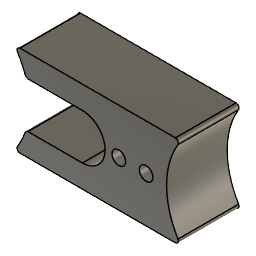
CUERPOMESA (Autodesk Fusion 360 design; units mm, degrees)
part number: 2026-05-18-09-44-16-687
Autodesk Fusion 360 part; units mm, degrees
sketch "Boceto2" plane through (0, 0, 0) normal (0, 1, 0) x (1, 0, 0)
  line L0 (-36.936, 0) -> (-1061.822, 0)
  line L1 (-1061.822, -600) -> (-36.936, -600)
  line L2 (-1008.5735, -150) -> (-650, -150)
  line L3 (-650, -450) -> (-1008.5735, -450)
  arc A0 (-1078.675, -569.2308) -> (-1027.4745, -463.4615) centre (-1500, -300) ccw
  arc A1 (-1027.4745, -136.5385) -> (-1078.675, -30.7692) centre (-1500, -300) ccw
  arc A2 (-650, -450) -> (-500, -300) centre (-650, -300) ccw
  arc A3 (-500, -300) -> (-650, -150) centre (-650, -300) ccw
  circle A4 centre (-410, -300) radius 45
  circle A5 centre (-230, -300) radius 45
  arc A6 (-19.821, -30.3477) -> (-19.821, -569.6523) centre (426.1842, -300) ccw
  arc A7 (-1078.675, -569.2308) -> (-1061.822, -600) centre (-1061.822, -580) ccw
  arc A8 (-36.936, -600) -> (-19.821, -569.6523) centre (-36.936, -580) ccw
  arc A9 (-19.821, -30.3477) -> (-36.936, 0) centre (-36.936, -20) ccw
  arc A10 (-1061.822, 0) -> (-1078.675, -30.7692) centre (-1061.822, -20) ccw
  arc A11 (-1027.4745, -136.5385) -> (-1008.5735, -150) centre (-1008.5735, -130) ccw
  arc A12 (-1008.5735, -450) -> (-1027.4745, -463.4615) centre (-1008.5735, -470) ccw
  point P0 (-1100, 0)
  point P1 (0, -600)
  point P2 (-500, -150)
  point P3 (-500, -450)
  dimension "d1" = 1100
  dimension "d2" = 600
  dimension "d6" = 300
  dimension "d13" = 150
  dimension "d14" = 150
  dimension "d15" = 90
  dimension "d16" = 90
  dimension "d17" = 180
  dimension "d18" = 90
  dimension "d20" = 20
  dimension "d21" = 20
  dimension "d22" = 20
  dimension "d23" = 20
  dimension "d24" = 20
  dimension "d25" = 20
  constraint horizontal L0
  constraint horizontal L1
  constraint concentric A0 A1
  constraint coincident P3 L3
  constraint tangent L3 A2
  constraint coincident P2 L2
  constraint tangent L2 A3
  constraint coincident A2.end A3.start
  constraint tangent L1 A7
  constraint tangent A0 A7
  constraint coincident P1 L1
  constraint coincident P1 A6
  constraint tangent A6 A8
  constraint tangent L1 A8
  constraint coincident origin L0
  constraint coincident origin A6
  constraint tangent A6 A9
  constraint tangent L0 A9
  constraint coincident P0 L0
  constraint coincident P0 A1
  constraint tangent L0 A10
  constraint tangent A1 A10
  constraint tangent L2 A11
  constraint tangent A1 A11
  constraint tangent L3 A12
  constraint tangent A0 A12
  measures "d1" distance of origin P0
  measures "d2" distance of origin P1
  measures "d6" distance of P2 P3
  measures "d13" radius of A2
  measures "d14" radius of A3
  measures "d15" distance of A2.end A4.centre
  measures "d16" diameter of A4
  measures "d17" distance of A4.centre A5.centre
  measures "d18" diameter of A5
  measures "d20" radius of A7
  measures "d21" radius of A8
  measures "d22" radius of A9
  measures "d23" radius of A10
  measures "d24" radius of A11
  measures "d25" radius of A12
extrude "Extruir1" add sketch "Boceto2" along normal blind 400
